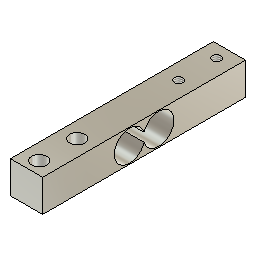
vibroDoser (Autodesk Fusion 360 archive; units mm, degrees)
design "LoadCell"
Autodesk Fusion 360 part; units mm, degrees
(part 1 of 2)
sketch "Skizze2" plane through (0, 0, 0) normal (0, 1, 0) x (1, 0, 0)
  line L0 (-6.35, -6.35) -> (6.35, -6.35)
  line L1 (6.35, -6.35) -> (6.35, 6.35)
  line L2 (6.35, 6.35) -> (-6.35, 6.35)
  line L3 (-6.35, 6.35) -> (-6.35, -6.35)
  line L4 (-6.35, -6.35) -> (6.35, 6.35) construction
  line L5 (6.35, -6.35) -> (-6.35, 6.35) construction
  dimension "d1" = 12.7
  dimension "d2" = 12.7
  constraint horizontal L0
  constraint perpendicular L0 L1
  constraint parallel L0 L2
  constraint parallel L1 L3
  constraint coincident L4 origin
  constraint coincident L5 origin
  measures "d1" distance of L1.end L2.end
  measures "d2" distance of L0.end L1.end
extrude "Extrusion1" add sketch "Skizze2" along normal blind 80
sketch "Skizze3" plane through (6.35, 0, 0) normal (1, 0, 0) x (0, 1, 0)
  line L0 (0, 6.35) -> (0, -6.35)
  line L1 (0, -6.35) -> (80, -6.35)
  line L2 (80, -6.35) -> (80, 6.35)
  line L3 (80, 6.35) -> (0, 6.35)
  line L4 (0, 0) -> (85.7645, 0) construction
  circle A0 centre (34.25, 0) radius 6
  circle A1 centre (45.75, 0) radius 6
  line L5 (40, -6.35) -> (40, 14.7485) construction
  dimension "d5" = 11.5
  dimension "d6" = 12
  dimension "d7" = 12
  dimension "d8" = 5.75
  constraint coincident L4.start origin
  constraint perpendicular L0 L4
  constraint coincident L4 A0.centre
  constraint coincident L4 A1.centre
  constraint midpoint L1 L5.start
  constraint perpendicular L3 L5
  measures "d5" distance of A0.centre A1.centre
  measures "d6" diameter of A1
  measures "d7" diameter of A0
  measures "d8" distance of A0.centre L5
extrude "Extrusion2" cut sketch "Skizze3" against normal blind 27 contours A0 A1 | A0 A1 | A0 A1
sketch "Skizze4" plane through (0, 0, 6.35) normal (0, 0, 1) x (-1, 0, 0)
  line L0 (6.35, 0) -> (-6.35, 0)
  line L1 (-6.35, 0) -> (-6.35, -80)
  line L2 (-6.35, -80) -> (6.35, -80)
  line L3 (6.35, -80) -> (6.35, 0)
  line L4 (0, 5.2844) -> (0, -87.2424)
  point P0 (0, -5)
  point P1 (0, -20)
  point P2 (0, -60)
  point P3 (0, -75)
  dimension "d11" = 5
  dimension "d12" = 15
  dimension "d13" = 15
  dimension "d14" = 5
  constraint perpendicular L2 L4
  constraint coincident origin L4
  constraint coincident L4 P0
  constraint coincident L4 P1
  constraint coincident L4 P2
  constraint coincident L4 P3
  measures "d11" distance of L0 P0
  measures "d12" distance of P0 P1
  measures "d13" distance of P2 P3
  measures "d14" distance of L2 P3
hole "Bohrung1" at (0, 5, 6.35) at (0, 20, 6.35) direction (0, 0, -1) diameter 6 depth 30 tip angle 118
hole "Bohrung2" at (0, 60, 6.35) at (0, 75, 6.35) direction (0, 0, -1) diameter 3.332 depth 30 tip angle 118
thread "Gewinde2" "ISO Metric profile 4.0 M4x0.7 6H"
equation "d8 = ( 11.5 / 2 ) * 1 mm"

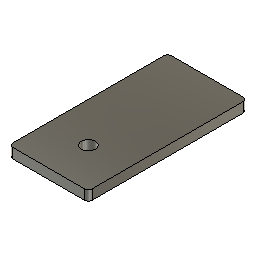
design "FussPlatte_4x"
Autodesk Fusion 360 part; units mm, degrees
sketch "Skizze1" plane through (0, 0, 0) normal (0, 0, 1) x (1, 0, 0)
  line L0 (-20, 40) -> (20, 40)
  line L1 (20, 40) -> (20, -40)
  line L2 (20, -40) -> (-20, -40)
  line L3 (-20, -40) -> (-20, 40)
  line L4 (-20, 40) -> (20, -40) construction
  line L5 (20, 40) -> (-20, -40) construction
  dimension "d1" = 40
  dimension "d2" = 80
  constraint horizontal L0
  constraint perpendicular L0 L1
  constraint parallel L0 L2
  constraint parallel L1 L3
  constraint coincident L4 origin
  constraint coincident L5 origin
  measures "d1" distance of L1.end L2.end
  measures "d2" distance of L0.end L1.end
extrude "Extrusion1" add sketch "Skizze1" along normal blind 5
sketch "Skizze2" plane through (0, 0, 5) normal (0, 0, 1) x (-1, 0, 0)
  line L0 (20, 40) -> (-20, 40)
  line L1 (-20, 40) -> (-20, -40)
  line L2 (-20, -40) -> (20, -40)
  line L3 (20, -40) -> (20, 40)
  line L4 (0, 0) -> (0, 20)
  dimension "d5" = 20
  constraint coincident L4.start origin
  constraint vertical L4
  measures "d5" distance of L0 L4.end
hole "Bohrung1" at (0, -20, 5) direction (0, 0, -1) diameter 7 depth 100 tip angle 118
fillet "Abrundung1" radius 2 4 edges at (-20, -40, 2.5) (20, -40, 2.5) (-20, 40, 2.5) (20, 40, 2.5)

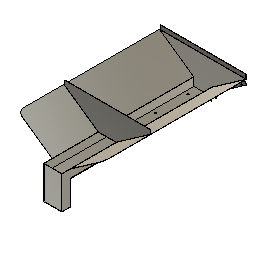
design "Rinne"
Autodesk Fusion 360 part; units mm, degrees
sketch "Skizze1" plane through (0, 0, 0) normal (0, 1, 0) x (1, 0, 0)
  line L0 (-33.75, -15.625) -> (33.75, -15.625)
  line L1 (33.75, -15.625) -> (33.75, 15.625)
  line L2 (33.75, 15.625) -> (-33.75, 15.625)
  line L3 (-33.75, 15.625) -> (-33.75, -15.625)
  line L4 (-33.75, -15.625) -> (33.75, 15.625) construction
  line L5 (33.75, -15.625) -> (-33.75, 15.625) construction
  line L6 (-32.5, 14.375) -> (32.5, 14.375)
  line L7 (32.5, 14.375) -> (32.5, -25.625)
  line L8 (32.5, -25.625) -> (-32.5, -25.625)
  line L9 (-32.5, -25.625) -> (-32.5, 14.375)
  dimension "d3" = 1.25
  dimension "d4" = 1.25
  dimension "d5" = 1.25
  dimension "d10" = 10
  dimension "d64" = 65
  dimension "d65" = 30
  constraint horizontal L0
  constraint perpendicular L0 L1
  constraint parallel L0 L2
  constraint parallel L1 L3
  constraint coincident L4 origin
  constraint coincident L5 origin
  constraint horizontal L6
  constraint vertical L7
  constraint horizontal L8
  constraint vertical L9
  measures "d3" distance of L3 L9
  measures "d4" distance of L1 L7
  measures "d5" distance of L2 L6
  measures "d10" distance of L0 L8
  measures "d64" distance of L7.end L8.end
  measures "d65" distance of L0 L6
extrude "Extrusion1" add sketch "Skizze1" along normal blind 520 contours L0 L1 L2 L3 L6 L7 L9 makes body 1
sketch "Skizze6" plane through (0, 520, 0) normal (0, 1, 0) x (-1, 0, 0)
  line L0 (-33.75, 15.625) -> (-159.6594, 103.7877)
  line L1 (-159.6594, 103.7877) -> (-159.2481, 104.375)
  line L2 (33.75, 15.625) -> (159.6594, 103.7877)
  line L3 (159.6594, 103.7877) -> (159.2481, 104.375)
  line L4 (159.2481, 104.375) -> (32.5, 15.625)
  line L5 (-32.5, 15.625) -> (-159.2481, 104.375)
  line L6 (-159.2481, 104.375) -> (159.2481, 104.375) construction
  line L7 (32.5, 15.625) -> (33.75, 15.625)
  line L8 (33.75, 15.625) -> (33.75, -15.625)
  line L9 (33.75, -15.625) -> (-33.75, -15.625)
  line L10 (-33.75, -15.625) -> (-33.75, 15.625)
  line L11 (-33.75, 15.625) -> (-32.5, 15.625)
  line L12 (-32.5, 15.625) -> (-32.5, -14.375)
  line L13 (-32.5, -14.375) -> (32.5, -14.375)
  line L14 (32.5, -14.375) -> (32.5, 15.625)
  dimension "d50" = 35
  dimension "d51" = 35
  dimension "d52" = 120
  constraint perpendicular L0 L1
  constraint perpendicular L2 L3
  constraint parallel L2 L4
  constraint parallel L0 L5
  constraint horizontal L6
  constraint coincident L2.start L7.end
  constraint coincident L4.end L7.start
  constraint coincident L5.start L11.end
  constraint coincident L0.start L10.end
  measures "d50" angle of L5 L6
  measures "d51" angle of L4 L6
  measures "d52" distance of L6 L9
extrude "Extrusion5" add sketch "Skizze6" against normal up to surface (520 mm away) contours L0 L1 L5 L11 | L2 L3 L4 L7 bodies 1
sketch "Skizze7" plane through (0, 520, 0) normal (0, 1, 0) x (-1, 0, 0)
  line L0 (32.5, 15.625) -> (32.5, -14.375)
  line L1 (32.5, -14.375) -> (-32.5, -14.375)
  line L2 (-32.5, -14.375) -> (-32.5, 15.625)
  line L3 (-33.75, 15.625) -> (-33.75, -15.625)
  line L4 (-33.75, -15.625) -> (33.75, -15.625)
  line L5 (33.75, -15.625) -> (33.75, 15.625)
  line L6 (-88.9851, 104.375) -> (159.6594, 104.375)
  line L7 (159.6594, 104.375) -> (159.6594, 103.7877)
  line L8 (-88.9851, 104.375) -> (-159.6583, 104.375)
  line L9 (-159.6583, 104.375) -> (-159.6594, 103.7877)
  line L10 (-32.5, 15.625) -> (-159.2481, 104.375)
  line L11 (-159.2481, 104.375) -> (-159.6594, 103.7877)
  line L12 (-159.6594, 103.7877) -> (-33.75, 15.625)
  line L13 (33.75, 15.625) -> (159.6594, 103.7877)
  line L14 (159.6594, 103.7877) -> (159.2481, 104.375)
  line L15 (159.2481, 104.375) -> (32.5, 15.625)
  constraint vertical L7
  constraint coincident L7.end L13.end
  constraint coincident L9.end L11.end
  constraint coincident L8 L10.end
  constraint coincident L6.start L8.start
  constraint parallel L6 L8
  constraint horizontal L6
extrude "Extrusion6" add sketch "Skizze7" along normal blind 1 bodies 1
sketch "Skizze11" plane through (0, 0, -14.375) normal (0, 0, 1) x (-1, 0, 0)
  line L0 (32.5, 0) -> (-32.5, 0)
  line L1 (-32.5, 0) -> (-32.5, -520)
  line L2 (-32.5, -520) -> (32.5, -520)
  line L3 (32.5, -520) -> (32.5, 0)
  line L4 (19, -365) -> (-19, -365)
  line L5 (-19, -365) -> (-19, -485)
  line L6 (-19, -485) -> (19, -485)
  line L7 (19, -485) -> (19, -365)
  line L8 (19, -365) -> (-19, -485) construction
  line L9 (-19, -365) -> (19, -485) construction
  line L10 (0, 0) -> (0, -850)
  line L11 (-33.75, -521) -> (33.75, -521)
  point P0 (0, -425)
  point P1 (19, -485)
  point P2 (-19, -485)
  point P3 (-19, -365)
  point P4 (19, -365)
  dimension "d69" = 120
  dimension "d70" = 38
  dimension "d75" = 96
  constraint horizontal L4
  constraint perpendicular L4 L5
  constraint parallel L4 L6
  constraint parallel L5 L7
  constraint coincident L8 P0
  constraint coincident L9 P0
  constraint coincident L10.start origin
  constraint perpendicular L0 L10
  constraint coincident P0 L10
  constraint coincident P1 L6.end
  constraint coincident P2 L5.end
  constraint coincident P3 L4.end
  constraint coincident P4 L4.start
  constraint midpoint P0 L10
  measures "d69" distance of P3 P2
  measures "d70" distance of P2 P1
  measures "d75" distance of P0 L11
hole "Bohrung2" at (-19, 485, -14.375) at (19, 485, -14.375) at (19, 365, -14.375) at (-19, 365, -14.375) direction (0, 0, -1) diameter 6.2 depth 200 tip angle 118 bodies 1
sketch "Skizze12" plane through (0, 521, 0) normal (0, 1, 0) x (-1, 0, 0)
  line L0 (159.6594, 104.375) -> (-159.6583, 104.375)
  line L1 (-159.6583, 104.375) -> (-159.6594, 103.7877)
  line L2 (-159.6594, 103.7877) -> (-33.75, 15.625)
  line L3 (-33.75, 15.625) -> (-33.75, -15.625)
  line L4 (-33.75, -15.625) -> (33.75, -15.625)
  line L5 (33.75, -15.625) -> (33.75, 15.625)
  line L6 (33.75, 15.625) -> (159.6594, 103.7877)
  line L7 (159.6594, 103.7877) -> (159.6594, 104.375)
  line L8 (-33.75, 13.625) -> (-48.75, 13.625)
  line L9 (-48.75, 13.625) -> (-48.75, -13.625)
  line L10 (-48.75, -13.625) -> (-33.75, -13.625)
  line L11 (-33.75, -13.625) -> (-33.75, 13.625)
  line L12 (33.75, -13.625) -> (48.75, -13.625)
  line L13 (48.75, -13.625) -> (48.75, 13.625)
  line L14 (48.75, 13.625) -> (33.75, 13.625)
  line L15 (33.75, 13.625) -> (33.75, -13.625)
  line L16 (-151.743, 98.2446) -> (-45.0241, 23.5192)
  line L17 (-45.0241, 23.5192) -> (-53.6277, 11.2319)
  line L18 (-53.6277, 11.2319) -> (-160.3467, 85.9573)
  line L19 (-160.3467, 85.9573) -> (-151.743, 98.2446)
  line L20 (46.0373, 24.2286) -> (151.7438, 98.2451)
  line L21 (151.7438, 98.2451) -> (160.3474, 85.9579)
  line L22 (160.3474, 85.9579) -> (54.6409, 11.9414)
  line L23 (54.6409, 11.9414) -> (46.0373, 24.2286)
  line L24 (-31.75, -15.625) -> (31.75, -15.625)
  line L25 (31.75, -15.625) -> (31.75, -30.625)
  line L26 (31.75, -30.625) -> (-31.75, -30.625)
  line L27 (-31.75, -30.625) -> (-31.75, -15.625)
  line L28 (-157.6583, 104.375) -> (157.6594, 104.375)
  line L29 (157.6594, 104.375) -> (157.6594, 119.2259)
  line L30 (157.6594, 119.2259) -> (-157.6583, 119.2259)
  line L31 (-157.6583, 119.2259) -> (-157.6583, 104.375)
  line L32 (-157.6583, 104.375) -> (112.3417, 104.375)
  dimension "d79" = 15
  dimension "d82" = 15
  dimension "d83" = 15
  dimension "d86" = 15
  dimension "d88" = 15
  dimension "d89" = 10
  dimension "d90" = 10
  dimension "d97" = 15
  dimension "d127" = 15
  dimension "d129" = 2
  dimension "d130" = 2
  dimension "d131" = 2
  dimension "d132" = 2
  dimension "d184" = 2
  dimension "d185" = 2
  constraint horizontal L8
  constraint vertical L9
  constraint horizontal L10
  constraint vertical L11
  constraint coincident L3 L8.start
  constraint horizontal L12
  constraint vertical L13
  constraint horizontal L14
  constraint vertical L15
  constraint coincident L5 L12.start
  constraint coincident L10.end L12
  constraint coincident L8.start L14
  constraint perpendicular L16 L17
  constraint parallel L16 L18
  constraint parallel L17 L19
  constraint coincident L2 L16.end
  constraint parallel L2 L16
  constraint perpendicular L20 L21
  constraint parallel L20 L22
  constraint parallel L21 L23
  constraint coincident L6 L20.end
  constraint parallel L6 L20
  constraint horizontal L24
  constraint vertical L25
  constraint horizontal L26
  constraint vertical L27
  constraint coincident L3.end L24
  constraint horizontal L28
  constraint vertical L29
  constraint horizontal L30
  constraint vertical L31
  constraint coincident L0 L28.start
  constraint horizontal L32
  measures "d79" distance of L9.end L10.end
  measures "d82" distance of L12.start L12.end
  measures "d83" distance of L16.start L18.end
  measures "d86" distance of L20.end L21.end
  measures "d88" distance of L5.end L23
  measures "d89" distance of L0.start L21
  measures "d90" distance of L0.end L19
  measures "d97" distance of L24.start L26.end
  measures "d127" distance of L8.start L16.end
  measures "d129" distance of L3.end L10
  measures "d130" distance of L3.end L27
  measures "d131" distance of L4.end L25
  measures "d132" distance of L2.end L8
  measures "d184" distance of L0.end L31
  measures "d185" distance of L0.start L29
extrude "Extrusion8" add sketch "Skizze12" along normal blind 1.25 separate body makes body 2
sketch "Skizze13" plane through (0, 521, 0) normal (0, 1, 0) x (-1, 0, 0)
  line L0 (33.75, -15.625) -> (33.75, -13.625)
  line L1 (33.75, 15.625) -> (46.0373, 24.2286)
  line L2 (159.6594, 103.7877) -> (159.6594, 104.375)
  line L3 (159.6594, 104.375) -> (157.6594, 104.375)
  line L4 (-159.6583, 104.375) -> (-159.6594, 103.7877)
  line L5 (-159.6594, 103.7877) -> (-151.743, 98.2446)
  line L6 (-33.75, 15.625) -> (-33.75, 13.625)
  line L7 (-33.75, -15.625) -> (-31.75, -15.625)
  line L8 (33.75, -13.625) -> (48.75, -13.625)
  line L9 (48.75, -13.625) -> (48.75, 13.625)
  line L10 (48.75, 13.625) -> (33.75, 13.625)
  line L11 (33.75, 13.625) -> (33.75, 15.625)
  line L12 (46.0373, 24.2286) -> (54.6409, 11.9414)
  line L13 (54.6409, 11.9414) -> (160.3474, 85.9579)
  line L14 (160.3474, 85.9579) -> (151.7438, 98.2451)
  line L15 (151.7438, 98.2451) -> (159.6594, 103.7877)
  line L16 (-151.743, 98.2446) -> (-160.3467, 85.9573)
  line L17 (-160.3467, 85.9573) -> (-53.6277, 11.2319)
  line L18 (-53.6277, 11.2319) -> (-45.0241, 23.5192)
  line L19 (-45.0241, 23.5192) -> (-33.75, 15.625)
  line L20 (-33.75, 13.625) -> (-48.75, 13.625)
  line L21 (-48.75, 13.625) -> (-48.75, -13.625)
  line L22 (-48.75, -13.625) -> (-33.75, -13.625)
  line L23 (-33.75, -13.625) -> (-33.75, -15.625)
  line L24 (-31.75, -15.625) -> (-31.75, -30.625)
  line L25 (-31.75, -30.625) -> (31.75, -30.625)
  line L26 (31.75, -30.625) -> (31.75, -15.625)
  line L27 (157.6594, 104.375) -> (157.6594, 119.2259)
  line L28 (157.6594, 119.2259) -> (-157.6583, 119.2259)
  line L29 (-157.6583, 119.2259) -> (-157.6583, 104.375)
  line L30 (-157.6583, 104.375) -> (-159.6583, 104.375)
  line L31 (31.75, -15.625) -> (33.75, -15.625)
sketch "Skizze17" plane through (0, 522.25, 0) normal (0, 1, 0) x (-1, 0, 0)
  line L0 (31.75, -15.625) -> (33.75, -15.625)
  line L1 (33.75, -15.625) -> (33.75, -13.625)
  line L2 (33.75, -13.625) -> (48.75, -13.625)
  line L3 (48.75, -13.625) -> (48.75, 13.625)
  line L4 (48.75, 13.625) -> (33.75, 13.625)
  line L5 (33.75, 13.625) -> (33.75, 15.625)
  line L6 (33.75, 15.625) -> (46.0373, 24.2286)
  line L7 (46.0373, 24.2286) -> (54.6409, 11.9414)
  line L8 (54.6409, 11.9414) -> (160.3474, 85.9579)
  line L9 (160.3474, 85.9579) -> (151.7438, 98.2451)
  line L10 (151.7438, 98.2451) -> (159.6594, 103.7877)
  line L11 (159.6594, 103.7877) -> (159.6594, 104.375)
  line L12 (159.6594, 104.375) -> (157.6594, 104.375)
  line L13 (-159.6583, 104.375) -> (-159.6594, 103.7877)
  line L14 (-159.6594, 103.7877) -> (-151.743, 98.2446)
  line L15 (-151.743, 98.2446) -> (-160.3467, 85.9573)
  line L16 (-160.3467, 85.9573) -> (-53.6277, 11.2319)
  line L17 (-53.6277, 11.2319) -> (-45.0241, 23.5192)
  line L18 (-45.0241, 23.5192) -> (-33.75, 15.625)
  line L19 (-33.75, 15.625) -> (-33.75, 13.625)
  line L20 (-33.75, 13.625) -> (-48.75, 13.625)
  line L21 (-48.75, 13.625) -> (-48.75, -13.625)
  line L22 (-48.75, -13.625) -> (-33.75, -13.625)
  line L23 (-33.75, -13.625) -> (-33.75, -15.625)
  line L24 (-33.75, -15.625) -> (-31.75, -15.625)
  line L25 (-31.75, -15.625) -> (-31.75, -30.625)
  line L26 (-31.75, -30.625) -> (31.75, -30.625)
  line L27 (31.75, -30.625) -> (31.75, -15.625)
  line L28 (-158.0524, 89.2339) -> (-51.3334, 14.5085)
  line L29 (-44.75, 13.625) -> (-44.75, -13.625)
  line L30 (-31.75, -26.625) -> (31.75, -26.625)
  line L31 (157.6594, 104.375) -> (157.6594, 119.2259)
  line L32 (157.6594, 119.2259) -> (-157.6583, 119.2259)
  line L33 (-157.6583, 119.2259) -> (-157.6583, 104.375)
  line L34 (-157.6583, 104.375) -> (-159.6583, 104.375)
  point P0 (-141.6693, 77.7624)
  point P1 (-104.6929, 51.8712)
  point P2 (-67.7165, 25.9801)
  point P3 (-44.75, 5.625)
  point P4 (-44.75, -5.625)
  point P5 (0, -26.625)
  point P6 (-19.75, -26.625)
  dimension "d133" = 4
  dimension "d134" = 4
  dimension "d135" = 4
  dimension "d136" = 20
  dimension "d137" = 20
  dimension "d138" = 12
  dimension "d139" = 8
  dimension "d140" = 8
  constraint coincident L15 L28.start
  constraint coincident L17 L28.end
  constraint perpendicular L17 L28
  constraint coincident L20 L29.start
  constraint coincident L22 L29.end
  constraint perpendicular L22 L29
  constraint coincident L25 L30.start
  constraint coincident L27 L30.end
  constraint perpendicular L27 L30
  constraint coincident L28 P0
  constraint midpoint L28 P1
  constraint coincident L28 P2
  constraint coincident L29 P3
  constraint coincident L29 P4
  constraint midpoint L30 P5
  constraint coincident L30 P6
  measures "d133" distance of L16 L28
  measures "d134" distance of L21 L29
  measures "d135" distance of L26 L30
  measures "d136" distance of L28.start P0
  measures "d137" distance of L28.end P2
  measures "d138" distance of L30.start P6
  measures "d139" distance of L22 P4
  measures "d140" distance of L20 P3
hole "Bohrung3" at (141.6693, 522.25, 77.7624) at (104.6929, 522.25, 51.8712) at (67.7165, 522.25, 25.9801) at (44.75, 522.25, 5.625) at (44.75, 522.25, -5.625) at (19.75, 522.25, -26.625) at (0, 522.25, -26.625) direction (0, -1, 0) diameter 4 depth 40 tip angle 118 bodies 2
fillet "Abrundung6" radius 1 12 edges at (-160.3474, 521.625, 85.9579) (-54.6409, 521.625, 11.9414) (-48.75, 521.625, 13.625) (-48.75, 521.625, -13.625) (-31.75, 521.625, -30.625) (31.75, 521.625, -30.625) (48.75, 521.625, -13.625) (48.75, 521.625, 13.625) (53.6277, 521.625, 11.2319) (160.3467, 521.625, 85.9573) (-157.6594, 521.625, 119.2259) (157.6583, 521.625, 119.2259) on bodies 2
sketch "Skizze14" plane through (0, 0, 0) normal (0, -1, 0) x (1, 0, 0)
  line L0 (-33.75, 15.625) -> (-33.75, -15.625)
  line L1 (-33.75, -15.625) -> (33.75, -15.625)
  line L2 (33.75, -15.625) -> (33.75, 15.625)
  line L3 (33.75, 15.625) -> (159.6594, 103.7877)
  line L4 (159.6594, 103.7877) -> (159.2481, 104.375)
  line L5 (159.2481, 104.375) -> (32.5, 15.625)
  line L6 (32.5, 15.625) -> (32.5, -14.375)
  line L7 (32.5, -14.375) -> (-32.5, -14.375)
  line L8 (-32.5, -14.375) -> (-32.5, 15.625)
  line L9 (-32.5, 15.625) -> (-159.2481, 104.375)
  line L10 (-159.2481, 104.375) -> (-159.6594, 103.7877)
  line L11 (-159.6594, 103.7877) -> (-33.75, 15.625)
  line L12 (-33.75, 15.625) -> (33.75, 15.625)
  line L13 (-159.2481, 104.375) -> (159.2481, 104.375)
  arc A0 (157.6583, 118.2259) -> (156.6583, 119.2259) centre (156.6583, 118.2259) ccw
  line L14 (157.6583, 118.2259) -> (157.6583, 104.375)
  line L15 (157.6583, 104.375) -> (159.6583, 104.375)
  line L16 (159.6583, 104.375) -> (159.6594, 103.7877)
  line L17 (159.6594, 103.7877) -> (151.743, 98.2446)
  line L18 (151.743, 98.2446) -> (159.7731, 86.7765)
  arc A1 (159.5275, 85.3838) -> (159.7731, 86.7765) centre (158.954, 86.2029) ccw
  line L19 (159.5275, 85.3838) -> (54.4469, 11.8055)
  arc A2 (53.0542, 12.0511) -> (54.4469, 11.8055) centre (53.8733, 12.6246) ccw
  line L20 (53.0542, 12.0511) -> (45.0241, 23.5192)
  line L21 (45.0241, 23.5192) -> (33.75, 15.625)
  line L22 (33.75, 15.625) -> (33.75, 13.625)
  line L23 (33.75, 13.625) -> (47.75, 13.625)
  arc A3 (48.75, 12.625) -> (47.75, 13.625) centre (47.75, 12.625) ccw
  line L24 (48.75, 12.625) -> (48.75, -12.625)
  arc A4 (47.75, -13.625) -> (48.75, -12.625) centre (47.75, -12.625) ccw
  line L25 (47.75, -13.625) -> (33.75, -13.625)
  line L26 (33.75, -13.625) -> (33.75, -15.625)
  line L27 (33.75, -15.625) -> (31.75, -15.625)
  line L28 (31.75, -15.625) -> (31.75, -29.625)
  arc A5 (30.75, -30.625) -> (31.75, -29.625) centre (30.75, -29.625) ccw
  line L29 (30.75, -30.625) -> (-30.75, -30.625)
  arc A6 (-31.75, -29.625) -> (-30.75, -30.625) centre (-30.75, -29.625) ccw
  line L30 (-31.75, -29.625) -> (-31.75, -15.625)
  line L31 (-31.75, -15.625) -> (-33.75, -15.625)
  line L32 (-33.75, -15.625) -> (-33.75, -13.625)
  line L33 (-33.75, -13.625) -> (-47.75, -13.625)
  arc A7 (-48.75, -12.625) -> (-47.75, -13.625) centre (-47.75, -12.625) ccw
  line L34 (-48.75, -12.625) -> (-48.75, 12.625)
  arc A8 (-47.75, 13.625) -> (-48.75, 12.625) centre (-47.75, 12.625) ccw
  line L35 (-47.75, 13.625) -> (-33.75, 13.625)
  line L36 (-33.75, 13.625) -> (-33.75, 15.625)
  line L37 (-33.75, 15.625) -> (-46.0373, 24.2286)
  line L38 (-46.0373, 24.2286) -> (-54.0674, 12.7605)
  arc A9 (-55.4601, 12.5149) -> (-54.0674, 12.7605) centre (-54.8865, 13.3341) ccw
  line L39 (-55.4601, 12.5149) -> (-159.5283, 85.3843)
  arc A10 (-159.7739, 86.777) -> (-159.5283, 85.3843) centre (-158.9547, 86.2034) ccw
  line L40 (-159.7739, 86.777) -> (-151.7438, 98.2451)
  line L41 (-151.7438, 98.2451) -> (-159.6594, 103.7877)
  line L42 (-159.6594, 103.7877) -> (-159.6594, 104.375)
  line L43 (-159.6594, 104.375) -> (-157.6594, 104.375)
  line L44 (-157.6594, 104.375) -> (-157.6594, 118.2259)
  arc A11 (-156.6594, 119.2259) -> (-157.6594, 118.2259) centre (-156.6594, 118.2259) ccw
  line L45 (-156.6594, 119.2259) -> (156.6583, 119.2259)
  circle A12 centre (19.75, -26.625) radius 2
  circle A13 centre (44.75, 5.625) radius 2
  circle A14 centre (104.6929, 51.8712) radius 2
  circle A15 centre (141.6693, 77.7624) radius 2
  circle A16 centre (67.7165, 25.9801) radius 2
  circle A17 centre (44.75, -5.625) radius 2
  circle A18 centre (0, -26.625) radius 2
  constraint coincident L0.start L11.end
  constraint coincident L2.end L3.start
  constraint coincident L9.end L10.start
  constraint coincident L4.end L5.start
extrude "Extrusion9" add sketch "Skizze14" along normal blind 1.2 from surface at -170 separate body contours L5 L9 L12 L13 L15 L43 | L13 A0 L14 L44 A11 L45 makes body 3
mirror "Spiegeln1" about plane through (0, 0, 0) normal (1, 0, 0) of "Bohrung3"
sketch "Skizze15" plane through (0, 0, -15.625) normal (0, 0, -1) x (1, 0, 0)
  circle A0 centre (19, -365) radius 3.1
  circle A1 centre (-19, -485) radius 3.1
  circle A2 centre (19, -485) radius 3.1
  circle A3 centre (-19, -365) radius 3.1
  line L0 (33.75, 0) -> (-33.75, 0)
  line L1 (-33.75, 0) -> (-33.75, -521)
  line L2 (-33.75, -521) -> (33.75, -521)
  line L3 (33.75, -521) -> (33.75, 0)
  line L4 (-33.75, -521) -> (-218.75, -521)
  line L5 (-218.75, -521) -> (-218.75, 0)
  line L6 (-218.75, 0) -> (-33.75, 0)
  line L7 (-33.75, 0) -> (-33.75, -521)
  line L8 (33.75, -521) -> (218.75, -521)
  line L9 (218.75, -521) -> (218.75, 0)
  line L10 (218.75, 0) -> (33.75, 0)
  line L11 (33.75, 0) -> (33.75, -521)
  circle A4 centre (19, -365) radius 3.1
  circle A5 centre (-19, -485) radius 3.1
  circle A6 centre (19, -485) radius 3.1
  circle A7 centre (-19, -365) radius 3.1
  line L12 (-32.5, 0) -> (32.5, 0)
  line L13 (32.5, 0) -> (32.5, -520)
  line L14 (32.5, -520) -> (-32.5, -520)
  line L15 (-32.5, -520) -> (-32.5, 0)
  line L16 (-33.75, 0) -> (33.75, 0)
  line L17 (33.75, 0) -> (33.75, 90)
  line L18 (33.75, 90) -> (-33.75, 90)
  line L19 (-33.75, 90) -> (-33.75, 0)
  dimension "d101" = 185
  dimension "d102" = 185
  dimension "d143" = 90
  constraint horizontal L4
  constraint vertical L5
  constraint horizontal L6
  constraint vertical L7
  constraint coincident L1.end L2.start
  constraint horizontal L8
  constraint vertical L9
  constraint horizontal L10
  constraint vertical L11
  constraint coincident L2.end L3.start
  constraint coincident L0.end L6
  constraint coincident L0.start L10
  constraint horizontal L16
  constraint vertical L17
  constraint horizontal L18
  constraint vertical L19
  constraint coincident L0.end L1.start
  constraint coincident L0.start L17
  measures "d101" distance of L1.end L4.end
  measures "d102" distance of L2.end L8.end
  measures "d143" distance of L0.start L17.end
extrude "Extrusion10" add sketch "Skizze15" along normal blind 1 separate body makes body 4
fillet "Abrundung5" radius 20 4 edges at (-159.4538, 0, 104.0813) (159.4538, 0, 104.0813) (-218.75, 0, -16.125) (218.75, 0, -16.125) on bodies 1 4
sketch "Skizze23" plane through (0, 0, 0) normal (0, -1, 0) x (1, 0, 0)
  line L0 (143.2763, 92.3162) -> (142.8651, 92.9035)
  line L1 (142.8651, 92.9035) -> (32.5, 15.625)
  line L2 (32.5, 15.625) -> (32.5, -14.375)
  line L3 (32.5, -14.375) -> (-32.5, -14.375)
  line L4 (-32.5, -14.375) -> (-32.5, 15.625)
  line L5 (-32.5, 15.625) -> (-142.8651, 92.9035)
  line L6 (-142.8651, 92.9035) -> (-143.2763, 92.3162)
  line L7 (-143.2763, 92.3162) -> (-33.75, 15.625)
  line L8 (-33.75, 15.625) -> (-33.75, -15.625)
  line L9 (-33.75, -15.625) -> (33.75, -15.625)
  line L10 (33.75, -15.625) -> (33.75, 15.625)
  line L11 (33.75, 15.625) -> (143.2763, 92.3162)
  line L12 (-33.75, 15.625) -> (33.75, 15.625)
  line L13 (-32.5, -14.375) -> (-32.5, -15.625)
  line L14 (32.5, -14.375) -> (32.5, -15.625)
  constraint coincident L7.end L8.start
  constraint coincident L10.end L11.start
  constraint coincident L3.end L4.start
  constraint coincident L9 L13.end
  constraint perpendicular L9 L13
  constraint coincident L2.end L3.start
  constraint coincident L9 L14.end
  constraint perpendicular L9 L14
extrude "Extrusion12" add sketch "Skizze23" along normal blind 30 contours L2 L9 L10 L12 L14 | L4 L8 L9 L12 L13 bodies 1
sketch "Skizze24" plane through (0, -30, 0) normal (0, -1, 0) x (1, 0, 0)
  line L0 (-33.75, 15.625) -> (-33.75, -15.625)
  line L1 (-33.75, -15.625) -> (-32.5, -15.625)
  line L2 (-32.5, -15.625) -> (-32.5, 15.625)
  line L3 (-32.5, 15.625) -> (-33.75, 15.625)
  line L4 (32.5, 15.625) -> (32.5, -15.625)
  line L5 (32.5, -15.625) -> (33.75, -15.625)
  line L6 (33.75, -15.625) -> (33.75, 15.625)
  line L7 (33.75, 15.625) -> (32.5, 15.625)
  line L8 (-33.75, 15.625) -> (33.75, 15.625)
  line L9 (33.75, 15.625) -> (33.75, -15.625)
  line L10 (33.75, -15.625) -> (-33.75, -15.625)
  line L11 (-33.75, -15.625) -> (-33.75, 15.625)
  constraint horizontal L8
  constraint vertical L9
  constraint horizontal L10
  constraint vertical L11
  constraint coincident L5.end L6.start
  constraint coincident L0.start L3.end
extrude "Extrusion13" add sketch "Skizze24" along normal blind 1.25 bodies 1
sketch "Skizze25" plane through (0, 0, -15.625) normal (0, 0, -1) x (1, 0, 0)
  line L0 (-33.75, 31.25) -> (-33.75, -521)
  line L1 (-33.75, -521) -> (33.75, -521)
  line L2 (33.75, -521) -> (33.75, 31.25)
  line L3 (33.75, 31.25) -> (-33.75, 31.25)
  circle A0 centre (19, -365) radius 3.1
  circle A1 centre (-19, -485) radius 3.1
  circle A2 centre (19, -485) radius 3.1
  circle A3 centre (-19, -365) radius 3.1
  line L4 (-32.5, 30) -> (32.5, 30)
  line L5 (32.5, 30) -> (32.5, 0)
  line L6 (32.5, 0) -> (-32.5, 0)
  line L7 (-32.5, 0) -> (-32.5, 30)
  line L8 (-33.75, 31.25) -> (33.75, 31.25)
  line L9 (33.75, 31.25) -> (33.75, -1.25)
  line L10 (33.75, -1.25) -> (-33.75, -1.25)
  line L11 (-33.75, -1.25) -> (-33.75, 31.25)
  dimension "d169" = 1.25
  constraint horizontal L8
  constraint vertical L9
  constraint horizontal L10
  constraint vertical L11
  constraint coincident L2 L9.end
  constraint coincident L0.start L3.end
  measures "d169" distance of L6 L10
extrude "Extrusion14" add sketch "Skizze25" along normal blind 90 contours L0 L2 L3 L8 L9 L10 L11 bodies 1
sketch "Skizze20" plane through (0, 0, -15.625) normal (0, 0, 1) x (-1, 0, 0)
  circle A0 centre (19, -365) radius 3.1
  circle A1 centre (-19, -485) radius 3.1
  circle A2 centre (-19, -365) radius 3.1
  circle A3 centre (19, -485) radius 3.1
  arc A4 (-198.75, 0) -> (-218.75, -20) centre (-198.75, -20) ccw
  line L0 (-218.75, -20) -> (-218.75, -521)
  line L1 (-218.75, -521) -> (218.75, -521)
  line L2 (218.75, -521) -> (218.75, -20)
  arc A5 (218.75, -20) -> (198.75, 0) centre (198.75, -20) ccw
  line L3 (198.75, 0) -> (33.75, 0)
  line L4 (33.75, 0) -> (33.75, 90)
  line L5 (33.75, 90) -> (-33.75, 90)
  line L6 (-33.75, 90) -> (-33.75, 0)
  line L7 (-33.75, 0) -> (-198.75, 0)
  line L8 (33.75, 140) -> (-33.75, 140)
  line L9 (-33.75, 140) -> (-33.75, 264)
  line L10 (-33.75, 264) -> (33.75, 264)
  line L11 (33.75, 264) -> (33.75, 140)
  line L12 (33.75, 140) -> (65.25, 140)
  line L13 (65.25, 140) -> (65.25, 264)
  line L14 (65.25, 264) -> (33.75, 264)
  line L15 (33.75, 264) -> (33.75, 140)
  line L16 (-33.75, 140) -> (-65.25, 140)
  line L17 (-65.25, 140) -> (-65.25, 264)
  line L18 (-65.25, 264) -> (-33.75, 264)
  line L19 (-33.75, 264) -> (-33.75, 140)
  line L20 (65.25, 142) -> (80.25, 142)
  line L21 (80.25, 142) -> (80.25, 262)
  line L22 (80.25, 262) -> (65.25, 262)
  line L23 (65.25, 262) -> (65.25, 142)
  line L24 (-65.25, 262) -> (-80.25, 262)
  line L25 (-80.25, 262) -> (-80.25, 142)
  line L26 (-80.25, 142) -> (-65.25, 142)
  line L27 (-65.25, 142) -> (-65.25, 262)
  line L28 (80.25, 172) -> (65.25, 172)
  line L29 (65.25, 172) -> (65.25, 174)
  line L30 (65.25, 174) -> (80.25, 174)
  line L31 (80.25, 174) -> (80.25, 172)
  line L32 (-65.25, 172) -> (-80.25, 172)
  line L33 (-80.25, 172) -> (-80.25, 174)
  line L34 (-80.25, 174) -> (-65.25, 174)
  line L35 (-65.25, 174) -> (-65.25, 172)
  dimension "d144" = 50
  dimension "d145" = 31.5
  dimension "d146" = 31.5
  dimension "d147" = 2
  dimension "d148" = 2
  dimension "d149" = 2
  dimension "d150" = 2
  dimension "d151" = 15
  dimension "d152" = 15
  dimension "d164" = 120
  dimension "d172" = 90
  dimension "d173" = 2
  dimension "d174" = 90
  dimension "d175" = 2
  constraint horizontal L8
  constraint vertical L9
  constraint horizontal L10
  constraint vertical L11
  constraint coincident L4.end L11
  constraint coincident L5.end L9
  constraint horizontal L12
  constraint vertical L13
  constraint horizontal L14
  constraint vertical L15
  constraint horizontal L16
  constraint vertical L17
  constraint horizontal L18
  constraint vertical L19
  constraint coincident L10.end L14
  constraint coincident L9.end L18
  constraint horizontal L20
  constraint vertical L21
  constraint horizontal L22
  constraint vertical L23
  constraint coincident L13 L20.start
  constraint horizontal L24
  constraint vertical L25
  constraint horizontal L26
  constraint vertical L27
  constraint coincident L17 L24.start
  constraint horizontal L28
  constraint vertical L29
  constraint horizontal L30
  constraint vertical L31
  constraint coincident L23 L29.end
  constraint coincident L21 L28.start
  constraint horizontal L32
  constraint vertical L33
  constraint horizontal L34
  constraint vertical L35
  constraint coincident L25 L33.end
  constraint coincident L17 L32.start
  measures "d144" distance of L5 L8
  measures "d145" distance of L8.start L12.end
  measures "d146" distance of L8.end L16.end
  measures "d147" distance of L12 L20
  measures "d148" distance of L16 L26
  measures "d149" distance of L14 L22
  measures "d150" distance of L18 L24
  measures "d151" distance of L24.start L24.end
  measures "d152" distance of L21.end L22.end
  measures "d164" distance of L24.end L25.end
  measures "d172" distance of L14 L30
  measures "d173" distance of L28 L30
  measures "d174" distance of L18 L34
  measures "d175" distance of L32 L34
extrude "Extrusion11" add sketch "Skizze20" along normal blind 1.25 separate body contours L8 L9 L10 L11 L15 L19 | L11 L12 L13 L14 L15 L23 L29 | L9 L16 L17 L18 L19 L27 L35 | L13 L20 L21 L23 L28 | L17 L25 L26 L27 L32 | L13 L21 L22 L23 L30 | L17 L24 L25 L27 L34 makes body 5
sketch "Skizze21" plane through (0, 0, -15.625) normal (0, 0, -1) x (1, 0, 0)
  line L0 (80.25, 262) -> (65.25, 262)
  line L1 (65.25, 262) -> (65.25, 264)
  line L2 (65.25, 264) -> (-65.25, 264)
  line L3 (-65.25, 264) -> (-65.25, 262)
  line L4 (-65.25, 262) -> (-80.25, 262)
  line L5 (-80.25, 262) -> (-80.25, 174)
  line L6 (-80.25, 142) -> (-65.25, 142)
  line L7 (-65.25, 142) -> (-65.25, 140)
  line L8 (-65.25, 140) -> (65.25, 140)
  line L9 (65.25, 140) -> (65.25, 142)
  line L10 (65.25, 142) -> (80.25, 142)
  line L11 (80.25, 142) -> (80.25, 172)
  line L12 (75.25, 142) -> (75.25, 262)
  line L13 (-75.25, 262) -> (-75.25, 142)
  line L14 (-80.25, 174) -> (-65.25, 174)
  line L15 (-65.25, 174) -> (-65.25, 172)
  line L16 (-65.25, 172) -> (-80.25, 172)
  line L17 (-80.25, 172) -> (-80.25, 142)
  line L18 (80.25, 172) -> (65.25, 172)
  line L19 (65.25, 172) -> (65.25, 174)
  line L20 (65.25, 174) -> (80.25, 174)
  line L21 (80.25, 174) -> (80.25, 262)
  point P0 (75.25, 186)
  point P1 (-75.25, 186)
  point P2 (-75.25, 148)
  point P3 (75.25, 148)
  point P4 (75.25, 250)
  point P5 (-75.25, 250)
  point P6 (-75.25, 166)
  point P7 (75.25, 166)
  dimension "d155" = 5
  dimension "d156" = 5
  dimension "d157" = 12
  dimension "d159" = 12
  dimension "d176" = 12
  dimension "d177" = 12
  dimension "d178" = 6
  dimension "d179" = 6
  dimension "d180" = 6
  dimension "d181" = 6
  constraint coincident L10 L12.start
  constraint coincident L0 L12.end
  constraint perpendicular L0 L12
  constraint coincident L4 L13.start
  constraint coincident L6 L13.end
  constraint perpendicular L6 L13
  constraint coincident L13 P2
  constraint coincident L12 P3
  constraint coincident L12 P4
  constraint coincident L13 P5
  constraint coincident L12 P0
  constraint coincident L13 P1
  constraint coincident L13 P6
  constraint coincident L12 P7
  measures "d155" distance of L11 L12
  measures "d156" distance of L5 L13
  measures "d157" distance of L0 P4
  measures "d159" distance of L4 P5
  measures "d176" distance of P1 L14
  measures "d177" distance of P0 L20
  measures "d178" distance of L6 P2
  measures "d179" distance of L10 P3
  measures "d180" distance of L16 P6
  measures "d181" distance of L18 P7
hole "Bohrung4" at (75.25, -250, -15.625) at (75.25, -186, -15.625) at (75.25, -148, -15.625) at (-75.25, -148, -15.625) at (-75.25, -186, -15.625) at (-75.25, -250, -15.625) at (-75.25, -166, -15.625) at (75.25, -166, -15.625) direction (0, 0, 1) diameter 4 depth 4 tip angle 118 bodies 5
sketch "Skizze22" plane through (0, 0, -14.375) normal (0, 0, 1) x (-1, 0, 0)
  circle A0 centre (75.25, 186) radius 2
  circle A1 centre (-75.25, 148) radius 2
  circle A2 centre (-75.25, 250) radius 2
  circle A3 centre (-75.25, 186) radius 2
  circle A4 centre (75.25, 148) radius 2
  circle A5 centre (75.25, 250) radius 2
  line L0 (-65.25, 262) -> (-80.25, 262)
  line L1 (-80.25, 262) -> (-80.25, 174)
  line L2 (-80.25, 142) -> (-65.25, 142)
  line L3 (-65.25, 174) -> (-65.25, 172)
  line L4 (-65.25, 140) -> (65.25, 140)
  line L5 (65.25, 140) -> (65.25, 142)
  line L6 (65.25, 142) -> (80.25, 142)
  line L7 (80.25, 142) -> (80.25, 172)
  line L8 (80.25, 262) -> (65.25, 262)
  line L9 (65.25, 172) -> (65.25, 174)
  line L10 (65.25, 264) -> (-65.25, 264)
  line L11 (-65.25, 264) -> (-65.25, 262)
  line L12 (-80.25, 174) -> (-65.25, 174)
  line L13 (-65.25, 172) -> (-80.25, 172)
  line L14 (-80.25, 172) -> (-80.25, 142)
  line L15 (80.25, 172) -> (65.25, 172)
  line L16 (65.25, 174) -> (80.25, 174)
  line L17 (80.25, 174) -> (80.25, 262)
  circle A6 centre (75.25, 166) radius 2
  circle A7 centre (-75.25, 166) radius 2
  line L18 (-65.25, 142) -> (-65.25, 140)
  line L19 (65.25, 262) -> (65.25, 264)
sketch "Skizze16" plane through (0, 0, -16.625) normal (0, 0, -1) x (1, 0, 0)
  arc A0 (218.75, -20) -> (198.75, 0) centre (198.75, -20) ccw
  line L0 (198.75, 0) -> (33.75, 0)
  arc A1 (-198.75, 0) -> (-218.75, -20) centre (-198.75, -20) ccw
  line L1 (-218.75, -20) -> (-218.75, -521)
  line L2 (-218.75, -521) -> (218.75, -521)
  line L3 (218.75, -521) -> (218.75, -20)
  circle A2 centre (19, -485) radius 3.1
  circle A3 centre (19, -365) radius 3.1
  circle A4 centre (-19, -365) radius 3.1
  circle A5 centre (-19, -485) radius 3.1
  line L4 (33.75, 0) -> (33.75, 90)
  line L5 (33.75, 90) -> (-33.75, 90)
  line L6 (-33.75, 90) -> (-33.75, 0)
  line L7 (-33.75, 0) -> (-198.75, 0)
sketch "Skizze18" plane through (0, 522.25, 0) normal (0, 1, 0) x (-1, 0, 0)
  arc A0 (-159.7731, 86.7765) -> (-159.5275, 85.3838) centre (-158.954, 86.2029) ccw
  line L0 (-159.5275, 85.3838) -> (-54.4469, 11.8055)
  arc A1 (-54.4469, 11.8055) -> (-53.0542, 12.0511) centre (-53.8733, 12.6246) ccw
  line L1 (-53.0542, 12.0511) -> (-45.0241, 23.5192)
  line L2 (-45.0241, 23.5192) -> (-33.75, 15.625)
  line L3 (-33.75, 15.625) -> (-33.75, 13.625)
  line L4 (-33.75, 13.625) -> (-47.75, 13.625)
  arc A2 (-47.75, 13.625) -> (-48.75, 12.625) centre (-47.75, 12.625) ccw
  line L5 (-48.75, 12.625) -> (-48.75, -12.625)
  arc A3 (-48.75, -12.625) -> (-47.75, -13.625) centre (-47.75, -12.625) ccw
  line L6 (-47.75, -13.625) -> (-33.75, -13.625)
  line L7 (-33.75, -13.625) -> (-33.75, -15.625)
  line L8 (-33.75, -15.625) -> (-31.75, -15.625)
  line L9 (-31.75, -15.625) -> (-31.75, -29.625)
  arc A4 (-31.75, -29.625) -> (-30.75, -30.625) centre (-30.75, -29.625) ccw
  line L10 (-30.75, -30.625) -> (30.75, -30.625)
  arc A5 (30.75, -30.625) -> (31.75, -29.625) centre (30.75, -29.625) ccw
  line L11 (31.75, -29.625) -> (31.75, -15.625)
  line L12 (31.75, -15.625) -> (33.75, -15.625)
  line L13 (33.75, -15.625) -> (33.75, -13.625)
  line L14 (33.75, -13.625) -> (47.75, -13.625)
  arc A6 (47.75, -13.625) -> (48.75, -12.625) centre (47.75, -12.625) ccw
  line L15 (48.75, -12.625) -> (48.75, 12.625)
  arc A7 (48.75, 12.625) -> (47.75, 13.625) centre (47.75, 12.625) ccw
  line L16 (47.75, 13.625) -> (33.75, 13.625)
  line L17 (33.75, 13.625) -> (33.75, 15.625)
  line L18 (33.75, 15.625) -> (46.0373, 24.2286)
  line L19 (46.0373, 24.2286) -> (54.0674, 12.7605)
  arc A8 (54.0674, 12.7605) -> (55.4601, 12.5149) centre (54.8865, 13.3341) ccw
  line L20 (55.4601, 12.5149) -> (159.5283, 85.3843)
  arc A9 (159.5283, 85.3843) -> (159.7739, 86.777) centre (158.9547, 86.2034) ccw
  line L21 (159.7739, 86.777) -> (151.7438, 98.2451)
  line L22 (151.7438, 98.2451) -> (159.6594, 103.7877)
  line L23 (159.6594, 103.7877) -> (159.6594, 104.375)
  line L24 (-157.6583, 104.375) -> (-159.6583, 104.375)
  line L25 (-159.6583, 104.375) -> (-159.6594, 103.7877)
  line L26 (-159.6594, 103.7877) -> (-151.743, 98.2446)
  line L27 (-151.743, 98.2446) -> (-159.7731, 86.7765)
  circle A10 centre (67.7165, 25.9801) radius 2
  circle A11 centre (44.75, -5.625) radius 2
  circle A12 centre (44.75, 5.625) radius 2
  circle A13 centre (19.75, -26.625) radius 2
  circle A14 centre (104.6929, 51.8712) radius 2
  circle A15 centre (141.6693, 77.7624) radius 2
  circle A16 centre (-19.75, -26.625) radius 2
  circle A17 centre (-44.75, 5.625) radius 2
  circle A18 centre (-104.6929, 51.8712) radius 2
  circle A19 centre (-141.6693, 77.7624) radius 2
  circle A20 centre (-67.7165, 25.9801) radius 2
  circle A21 centre (-44.75, -5.625) radius 2
  circle A22 centre (0, -26.625) radius 2
  arc A23 (-156.6583, 119.2259) -> (-157.6583, 118.2259) centre (-156.6583, 118.2259) ccw
  line L28 (-157.6583, 118.2259) -> (-157.6583, 104.375)
  line L29 (159.6594, 104.375) -> (157.6594, 104.375)
  line L30 (157.6594, 104.375) -> (157.6594, 118.2259)
  arc A24 (157.6594, 118.2259) -> (156.6594, 119.2259) centre (156.6594, 118.2259) ccw
  line L31 (156.6594, 119.2259) -> (-156.6583, 119.2259)
hidden bodies 4 5

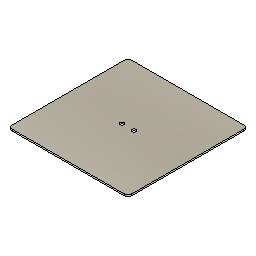
design "WiegeFläche1Cell"
Autodesk Fusion 360 part; units mm, degrees
sketch "Skizze1" plane through (0, 0, 0) normal (0, 0, 1) x (1, 0, 0)
  line L0 (-75, 75) -> (75, 75)
  line L1 (75, 75) -> (75, -75)
  line L2 (75, -75) -> (-75, -75)
  line L3 (-75, -75) -> (-75, 75)
  line L4 (-75, 75) -> (75, -75) construction
  line L5 (75, 75) -> (-75, -75) construction
  dimension "d1" = 150
  dimension "d2" = 150
  constraint horizontal L0
  constraint perpendicular L0 L1
  constraint parallel L0 L2
  constraint parallel L1 L3
  constraint coincident L4 origin
  constraint coincident L5 origin
  measures "d1" distance of L1.end L2.end
  measures "d2" distance of L0.end L1.end
extrude "Extrusion1" add sketch "Skizze1" along normal blind 2
fillet "Abrundung1" radius 5 4 edges at (75, -75, 1) (-75, -75, 1) (75, 75, 1) (-75, 75, 1)
sketch "Skizze3" plane through (0, 0, 2) normal (0, 0, 1) x (-1, 0, 0)
  arc A0 (70, -75) -> (75, -70) centre (70, -70) ccw
  line L0 (75, -70) -> (75, 70)
  line L1 (-75, 70) -> (-75, -70)
  line L2 (-70, -75) -> (70, -75)
  line L3 (7.5, 0) -> (-7.5, 0)
  dimension "d17" = 15
  dimension "d19" = 7.5
  constraint horizontal L3
  constraint coincident origin L3
  measures "d17" distance of L3.start L3.end
  measures "d19" distance of origin L3.start
hole "Bohrung1" at (7.5, 0, 2) at (-7.5, 0, 2) direction (0, 0, -1) diameter 5 depth 10 tip angle 118

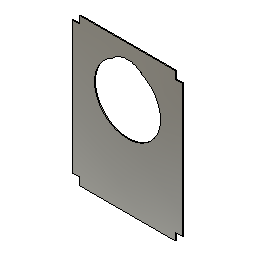
design "AufnahmePlatteTrichterGroß"
Autodesk Fusion 360 part; units mm, degrees
sketch "Skizze1" plane through (0, 0, 0) normal (0, 1, 0) x (1, 0, 0)
  line L0 (-300, 400) -> (300, 400)
  line L1 (300, 400) -> (300, -400)
  line L2 (300, -400) -> (-300, -400)
  line L3 (-300, -400) -> (-300, 400)
  line L4 (-300, 400) -> (300, -400) construction
  line L5 (300, 400) -> (-300, -400) construction
  line L6 (0, 273.6534) -> (0, -137.7109) construction
  circle A0 centre (0, -130) radius 179
  line L7 (-300, -400) -> (-259.5, -400)
  line L8 (-259.5, -400) -> (-259.5, -359.5)
  line L9 (-259.5, -359.5) -> (-300, -359.5)
  line L10 (-300, -359.5) -> (-300, -400)
  line L11 (-300, 400) -> (-259.5, 400)
  line L12 (-259.5, 400) -> (-259.5, 359.5)
  line L13 (-259.5, 359.5) -> (-300, 359.5)
  line L14 (-300, 359.5) -> (-300, 400)
  line L15 (300, 400) -> (259.5, 400)
  line L16 (259.5, 400) -> (259.5, 359.5)
  line L17 (259.5, 359.5) -> (300, 359.5)
  line L18 (300, 359.5) -> (300, 400)
  line L19 (300, -400) -> (259.5, -400)
  line L20 (259.5, -400) -> (259.5, -359.5)
  line L21 (259.5, -359.5) -> (300, -359.5)
  line L22 (300, -359.5) -> (300, -400)
  dimension "d1" = 600
  dimension "d2" = 800
  dimension "d7" = 358
  dimension "d22" = 270
  dimension "d38" = 40.5
  dimension "d39" = 40.5
  constraint horizontal L0
  constraint perpendicular L0 L1
  constraint parallel L0 L2
  constraint parallel L1 L3
  constraint coincident L4 origin
  constraint coincident L5 origin
  constraint vertical L6
  constraint coincident origin L6
  constraint coincident L6 A0.centre
  constraint horizontal L7
  constraint vertical L8
  constraint horizontal L9
  constraint vertical L10
  constraint horizontal L11
  constraint vertical L12
  constraint horizontal L13
  constraint vertical L14
  constraint horizontal L15
  constraint vertical L16
  constraint horizontal L17
  constraint vertical L18
  constraint horizontal L19
  constraint vertical L20
  constraint horizontal L21
  constraint vertical L22
  constraint equal L17 L21
  constraint equal L16 L17
  constraint equal L12 L16
  constraint equal L12 L13
  constraint equal L9 L12
  constraint equal L8 L9
  measures "d1" distance of L1.end L2.end
  measures "d2" distance of L0.end L1.end
  measures "d7" diameter of A0
  measures "d22" distance of L2 A0.centre
  measures "d38" distance of L1.end L19.end
  measures "d39" distance of L1.end L21.end
extrude "Extrusion1" add sketch "Skizze1" along normal blind 5 contours L0 L1 L2 L3 L8 L9 L12 L13 L16 L17 L20 L21
sketch "Skizze3" plane through (0, 0, 0) normal (0, -1, 0) x (1, 0, 0)
  circle A0 centre (0, 130) radius 179
  line L0 (259.5, 400) -> (-259.5, 400)
  line L1 (-300, 359.5) -> (-300, -359.5)
  line L2 (-259.5, -400) -> (259.5, -400)
  line L3 (300, -359.5) -> (300, 359.5)
  circle A1 centre (0, 130) radius 179
  line L4 (-75, 312.5) -> (75, 312.5)
  line L5 (75, 312.5) -> (75, -52.5)
  line L6 (75, -52.5) -> (-75, -52.5)
  line L7 (-75, -52.5) -> (-75, 312.5)
  line L8 (-75, 312.5) -> (75, -52.5) construction
  line L9 (75, 312.5) -> (-75, -52.5) construction
  circle A2 centre (0, 130) radius 182.5
  line L10 (-25, 322.5) -> (25, 322.5)
  line L11 (25, 322.5) -> (25, -62.5)
  line L12 (25, -62.5) -> (-25, -62.5)
  line L13 (-25, -62.5) -> (-25, 322.5)
  line L14 (-25, 322.5) -> (25, -62.5) construction
  line L15 (25, 322.5) -> (-25, -62.5) construction
  circle A3 centre (0, 201.7754) radius 120.7246
  line L16 (259.5, 359.5) -> (259.5, 400)
  line L17 (-259.5, 400) -> (-259.5, 359.5)
  line L18 (-259.5, 359.5) -> (-300, 359.5)
  line L19 (-300, -359.5) -> (-259.5, -359.5)
  line L20 (-259.5, -359.5) -> (-259.5, -400)
  line L21 (259.5, -400) -> (259.5, -359.5)
  line L22 (259.5, -359.5) -> (300, -359.5)
  line L23 (300, 359.5) -> (259.5, 359.5)
  point P0 (0, 130)
  point P1 (0, 130)
  point P2 (-75, 296.3768)
  point P3 (75, 296.3768)
  dimension "d30" = 150
  dimension "d31" = 365
  dimension "d32" = 50
  dimension "d33" = 10
  constraint horizontal L4
  constraint perpendicular L4 L5
  constraint parallel L4 L6
  constraint parallel L5 L7
  constraint coincident L8 P1
  constraint coincident L9 P1
  constraint coincident P1 P0
  constraint tangent L4 A2
  constraint horizontal L10
  constraint perpendicular L10 L11
  constraint parallel L10 L12
  constraint parallel L11 L13
  constraint coincident L14 P1
  constraint coincident L15 P1
  constraint tangent L10 A3
  constraint coincident L7 P2
  constraint coincident A2 P2
  constraint coincident L5 P3
  constraint coincident A2 P3
  constraint coincident A3 P2
  constraint coincident A3 P3
  measures "d30" distance of L4.start L4.end
  measures "d31" diameter of A2
  measures "d32" distance of L10.start L10.end
  measures "d33" distance of L4 L10
extrude "Extrusion2" cut sketch "Skizze3" against normal blind 20 contours A0 A1 L5 A2 L11 | L4 A2 L11 A3 | A0 A1 A2 L11 L13 | L4 A2 L11 | L4 L11 A3 | A0 A1 L7 A2 L13 | L4 A2 L13 | L4 L11 L13 A3 | L10 L11 A3 | L4 A2 L13 A3 | L4 L13 A3 | L10 L13 A3 picked at (69.6128, 295.9867) picked at (0, 310.0365) picked at (-69.6128, 295.9867)
fillet "Abrundung2" radius 2 8 edges at (-75, 2.5, 292.53) (-25, 2.5, 322.5) (25, 2.5, 322.5) (75, 2.5, 292.53) (-25, 2.5, 319.8831) (25, 2.5, 319.8831) (75, 2.5, 296.3768) (-75, 2.5, 296.3768)
fillet "Abrundung3" radius 2 12 edges at (-300, 2.5, -359.5) (-259.5, 2.5, -359.5) (-259.5, 2.5, -400) (259.5, 2.5, -400) (259.5, 2.5, -359.5) (300, 2.5, -359.5) (-300, 2.5, 359.5) (-259.5, 2.5, 359.5) (-259.5, 2.5, 400) (259.5, 2.5, 400) (259.5, 2.5, 359.5) (300, 2.5, 359.5)
sketch "Skizze4" plane through (0, 0, 0) normal (0, -1, 0) x (1, 0, 0)
  arc A0 (75, 293.8048) -> (76.1492, 291.9948) centre (77, 293.8048) ccw
  arc A1 (-76.1492, 291.9948) -> (76.1492, 291.9948) centre (0, 130) ccw
  arc A2 (-76.1492, 291.9948) -> (-75, 293.8048) centre (-77, 293.8048) ccw
  arc A3 (-23.1252, 322.5) -> (-25.0626, 320.9965) centre (-23.1252, 320.5) ccw
  line L0 (-23.1252, 322.5) -> (23.1252, 322.5)
  arc A4 (25.0626, 320.9965) -> (23.1252, 322.5) centre (23.1252, 320.5) ccw
  line L1 (257.5, 400) -> (-257.5, 400)
  line L2 (-300, 357.5) -> (-300, -357.5)
  line L3 (-257.5, -400) -> (257.5, -400)
  line L4 (300, -357.5) -> (300, 357.5)
  line L5 (-75, 293.8048) -> (-75, 295.4052)
  line L6 (75, 295.4052) -> (75, 293.8048)
  arc A5 (-26.56, 319.5421) -> (-74.2297, 296.9824) centre (0, 201.7754) ccw
  arc A6 (74.2297, 296.9824) -> (26.56, 319.5421) centre (0, 201.7754) ccw
  arc A7 (25.0626, 320.9965) -> (26.56, 319.5421) centre (27, 321.4931) ccw
  arc A8 (75, 295.4052) -> (74.2297, 296.9824) centre (73, 295.4052) ccw
  arc A9 (-74.2297, 296.9824) -> (-75, 295.4052) centre (-73, 295.4052) ccw
  arc A10 (-26.56, 319.5421) -> (-25.0626, 320.9965) centre (-27, 321.4931) ccw
  line L7 (259.5, 361.5) -> (259.5, 398)
  line L8 (-259.5, 398) -> (-259.5, 361.5)
  line L9 (-261.5, 359.5) -> (-298, 359.5)
  line L10 (-298, -359.5) -> (-261.5, -359.5)
  line L11 (-259.5, -361.5) -> (-259.5, -398)
  line L12 (259.5, -398) -> (259.5, -361.5)
  line L13 (261.5, -359.5) -> (298, -359.5)
  line L14 (298, 359.5) -> (261.5, 359.5)
  arc A11 (300, 357.5) -> (298, 359.5) centre (298, 357.5) ccw
  arc A12 (259.5, 361.5) -> (261.5, 359.5) centre (261.5, 361.5) ccw
  arc A13 (259.5, 398) -> (257.5, 400) centre (257.5, 398) ccw
  arc A14 (-257.5, 400) -> (-259.5, 398) centre (-257.5, 398) ccw
  arc A15 (-261.5, 359.5) -> (-259.5, 361.5) centre (-261.5, 361.5) ccw
  arc A16 (-298, 359.5) -> (-300, 357.5) centre (-298, 357.5) ccw
  arc A17 (-300, -357.5) -> (-298, -359.5) centre (-298, -357.5) ccw
  arc A18 (-259.5, -361.5) -> (-261.5, -359.5) centre (-261.5, -361.5) ccw
  arc A19 (-259.5, -398) -> (-257.5, -400) centre (-257.5, -398) ccw
  arc A20 (257.5, -400) -> (259.5, -398) centre (257.5, -398) ccw
  arc A21 (261.5, -359.5) -> (259.5, -361.5) centre (261.5, -361.5) ccw
  arc A22 (298, -359.5) -> (300, -357.5) centre (298, -357.5) ccw

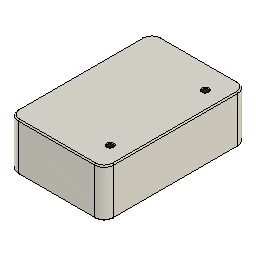
design "Schaltschrank"
Autodesk Fusion 360 part; units mm, degrees